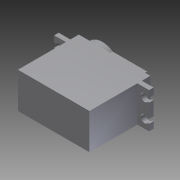
# Autodesk Inventor part: 7955
Saved by Autodesk Inventor 2012 (Build 160160000, 160)
## iProperties
Created: 2011-10-02
Part Number: 7955
Material: Default
Document SubType Name: Modeling
Designer: Yadi Irawan
Density: 1 g/cm^3
Author: Yadi Irawan
Autodesk Inventor part; units mm, degrees
ref_plane "YZ Plane" through (0, 0, 0) normal (1, 0, 0) x (0, 1, 0)
ref_plane "XZ Plane" through (0, 0, 0) normal (0, 1, 0) x (-1, 0, 0)
ref_plane "XY Plane" through (0, 0, 0) normal (0, 0, 1) x (1, 0, 0)
sketch "Sketch1" plane through (0, 0, 0) normal (0, 0, 1) x (1, 0, 0)
  line L0 (0, 0) -> (39.7, 0)
  line L1 (39.7, 0) -> (39.7, -37)
  line L2 (39.7, -37) -> (0, -37)
  line L3 (0, -37) -> (0, 0)
  dimension "d0" = 39.7
  dimension "d1" = 37
  constraints: 8 end point
  measures "d0" distance of L0.start L0.end
  measures "d1" distance of L0.end L1.end
extrude "Extrusion1" add sketch "Sketch1" along normal blind 19.8
sketch "Sketch2" plane through (39.7, -37, 0) normal (1, 0, 0) x (0, 0, -1)
  line L0 (-19.8, 37) -> (-19.8, 0) projected
  line L1 (0, 37) -> (0, 0) projected
  line L2 (0, 37) -> (-19.8, 37) projected
  line L3 (-19.8, 29.1) -> (0, 29.1)
  line L4 (0, 29.1) -> (0, 26.6)
  line L5 (0, 26.6) -> (-19.8, 26.6)
  line L6 (-19.8, 26.6) -> (-19.8, 29.1)
  dimension "d4" = 2.5
  dimension "d5" = 10.4
  constraints: 8 end point, 2 point on line
  measures "d4" distance of L5.end L3.start
  measures "d5" distance between parallel lines of L5 L2
extrude "Extrusion2" add sketch "Sketch2" along normal blind 6.5 contours L3 L1 L5 L0
sketch "Sketch3" plane through (39.7, -7.9, 19.8) normal (0, 1, 0) x (1, 0, 0)
  line L0 (6.5, 0) -> (6.5, 19.8) projected
  arc A0 (5.744, 16.2) -> (5.744, 13.8) centre (3.96, 15) ccw
  arc A1 (5.744, 6) -> (5.744, 3.6) centre (3.96, 4.8) ccw
  line L1 (6.5, 4.8) -> (6.5, 6)
  line L2 (6.5, 6) -> (5.744, 6)
  line L3 (6.5, 3.6) -> (5.744, 3.6)
  line L4 (6.5, 4.8) -> (6.5, 3.6)
  line L5 (6.5, 15) -> (6.5, 13.8)
  line L6 (6.5, 13.8) -> (5.744, 13.8)
  line L7 (5.744, 16.2) -> (6.5, 16.2)
  line L8 (6.5, 16.2) -> (6.5, 15)
  point P0 (-39.7, 19.8)
  constraints: 16 end point, 6 point on line, 4 point on circle, 2 centre point
extrude "Extrusion3" cut sketch "Sketch3" against normal blind 6.5
sketch "Sketch4" plane through (0, -37, 0) normal (-1, 0, 0) x (0, 0, 1)
  line L0 (19.8, 0) -> (19.8, 37) projected
  line L1 (0, 37) -> (19.8, 37) projected
  line L2 (0, 0) -> (0, 37) projected
  line L3 (0, 29.1) -> (19.8, 29.1)
  line L4 (19.8, 29.1) -> (19.8, 26.6)
  line L5 (19.8, 26.6) -> (0, 26.6)
  line L6 (0, 26.6) -> (0, 29.1)
  dimension "d18" = 2.5
  dimension "d19" = 10.4
  constraints: 8 end point, 2 point on line
  measures "d18" distance of L5.end L3.start
  measures "d19" distance between parallel lines of L5 L1
extrude "Extrusion4" add sketch "Sketch4" along normal blind 6.5 contours L5 L2 L3 L0
sketch "Sketch5" plane through (0, -7.9, 19.8) normal (0, 1, 0) x (1, 0, 0)
  line L0 (-6.5, 19.8) -> (-6.5, 0) projected
  arc A0 (-5.744, 3.6) -> (-5.744, 6) centre (-3.96, 4.8) ccw
  arc A1 (-5.744, 13.8) -> (-5.744, 16.2) centre (-3.96, 15) ccw
  line L1 (-6.5, 15) -> (-6.5, 16.2)
  line L2 (-6.5, 16.2) -> (-5.744, 16.2)
  line L3 (-5.744, 13.8) -> (-6.5, 13.8)
  line L4 (-6.5, 13.8) -> (-6.5, 15)
  line L5 (-6.5, 4.8) -> (-6.5, 6)
  line L6 (-6.5, 6) -> (-5.744, 6)
  line L7 (-5.744, 3.6) -> (-6.5, 3.6)
  line L8 (-6.5, 3.6) -> (-6.5, 4.8)
  dimension "d25" = 4.3
  dimension "d26" = 1.2
  dimension "d27" = 2.4
  constraints: 16 end point, 6 point on line, 4 point on circle, 2 centre point
  measures "d25" diameter of A0
  measures "d26" distance of L1.start L1.end
  measures "d27" distance of L6.end L7.start
extrude "Extrusion5" cut sketch "Sketch5" against normal blind 6.5
sketch "Sketch6" plane through (0, 0, 0) normal (0, 1, 0) x (1, 0, 0)
  line L0 (0, 0) -> (39.7, 0) projected
  line L1 (0, 0) -> (0, -19.8) projected
  circle A0 centre (9.9, -9.9) radius 2.5
  dimension "d30" = 5
  dimension "d31" = 19.8
  dimension "d32" = 9.9
  dimension "d33" = 9.9
  constraints: 1 centre point
  measures "d30" diameter of A0
  measures "d31" distance of L0.start L1.end
  measures "d32" distance from line of L0 A0.centre
  measures "d33" distance from line of L1 A0.centre
extrude "Extrusion6" add sketch "Sketch6" along normal blind 3.3
sketch "Sketch7" plane through (0, 0, 0) normal (0, 1, 0) x (1, 0, 0)
  circle A0 centre (9.9, -9.9) radius 2.5 projected
  line L0 (0, -19.8) -> (39.7, -19.8) projected
  line L1 (39.7, 0) -> (39.7, -19.8) projected
  line L2 (0, 0) -> (39.7, 0) projected
  line L3 (0, 0) -> (0, -19.8) projected
  arc A1 (15.5921, -2) -> (15.5921, -17.8) centre (9.9, -9.9) ccw
  line L4 (34.8, -2) -> (15.5921, -2)
  line L5 (34.8, -17.8) -> (15.5921, -17.8)
  arc A2 (34.8, -12.4) -> (34.8, -7.4) centre (34.8, -9.9) ccw
  line L6 (34.8, -2) -> (34.8, -7.4)
  line L7 (34.8, -12.4) -> (34.8, -17.8)
  dimension "d36" = 2
  dimension "d37" = 2
  dimension "d39" = 5
  constraints: 8 end point, 4 point on circle, 2 centre point, 1 coincident
  measures "d36" distance between parallel lines of L4 L2
  measures "d37" distance between parallel lines of L0 L5
  measures "d39" diameter of A2
extrude "Extrusion7" cut sketch "Sketch7" against normal blind 3.2 contours L3 L2 L1 L0
body "Solid1"
